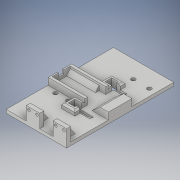
# Autodesk Inventor part: Elevator Slide
Saved by Autodesk Inventor 2018 (Build 220112000, 112)
## iProperties
Created: 2017-10-23
Part Number: Elevator Slide
Material: Generic
Document SubType Name: Modeling
Designer: thompson.nathaniel
Density: 1 g/cm^3
Appearance: Default
Author: thompson.nathaniel
Autodesk Inventor part; units mm, degrees
ref_plane "YZ Plane" through (0, 0, 0) normal (1, 0, 0) x (0, 1, 0)
ref_plane "XZ Plane" through (0, 0, 0) normal (0, 1, 0) x (-1, 0, 0)
ref_plane "XY Plane" through (0, 0, 0) normal (0, 0, 1) x (1, 0, 0)
sketch "Sketch1" plane through (0, 0, 0) normal (0, 1, 0) x (-1, 0, 0)
  line L0 (0, 0) -> (-114.3, 0)
  line L1 (-114.3, 0) -> (-114.3, 152.4)
  line L2 (-114.3, 152.4) -> (0, 152.4)
  line L3 (0, 152.4) -> (0, 0)
  line L4 (-69.85, 34.925) -> (-57.15, 34.925)
  line L5 (-57.15, 34.925) -> (-57.15, 47.625)
  line L6 (-57.15, 47.625) -> (-69.85, 47.625)
  line L7 (-69.85, 47.625) -> (-69.85, 34.925)
  line L8 (-69.85, 104.775) -> (-57.15, 104.775)
  line L9 (-57.15, 104.775) -> (-57.15, 117.475)
  line L10 (-57.15, 117.475) -> (-69.85, 117.475)
  line L11 (-69.85, 117.475) -> (-69.85, 104.775)
  dimension "d0" = 152.4
  dimension "d1" = 114.3
  dimension "d2" = 44.45
  dimension "d3" = 44.45
  dimension "d4" = 12.7
  dimension "d5" = 12.7
  dimension "d6" = 12.7
  dimension "d7" = 12.7
  dimension "d8" = 57.15
  dimension "d9" = 34.925
  constraints: 24 end point, 6 parallel, 3 horizontal, 3 perpendicular
  measures "d0" distance of L0.end L1.end
  measures "d1" distance of L0.start L0.end
  measures "d2" distance between parallel lines of L1 L7
  measures "d3" distance between parallel lines of L1 L11
  measures "d4" distance of L8.start L8.end
  measures "d5" distance of L10.end L8.start
  measures "d6" distance of L6.end L4.start
  measures "d7" distance of L4.start L4.end
  measures "d8" distance between parallel lines of L8 L6
  measures "d9" distance between parallel lines of L2 L10
extrude "Extrusion1" add sketch "Sketch1" along normal blind 10.16
sketch "Sketch2" plane through (0, 10.16, 0) normal (0, 1, 0) x (1, 0, 0)
  line L0 (50.8, -28.575) -> (76.2, -28.575)
  line L1 (76.2, -28.575) -> (76.2, -53.975)
  line L2 (76.2, -53.975) -> (50.8, -53.975)
  line L3 (50.8, -53.975) -> (50.8, -28.575)
  line L4 (50.8, -98.425) -> (76.2, -98.425)
  line L5 (76.2, -98.425) -> (76.2, -123.825)
  line L6 (76.2, -123.825) -> (50.8, -123.825)
  line L7 (50.8, -123.825) -> (50.8, -98.425)
  line L8 (57.15, -34.925) -> (69.85, -34.925) projected
  line L9 (69.85, -34.925) -> (69.85, -47.625) projected
  line L10 (69.85, -47.625) -> (57.15, -47.625) projected
  line L11 (57.15, -47.625) -> (57.15, -34.925) projected
  line L12 (57.15, -104.775) -> (69.85, -104.775) projected
  line L13 (69.85, -104.775) -> (69.85, -117.475) projected
  line L14 (69.85, -117.475) -> (57.15, -117.475) projected
  line L15 (57.15, -117.475) -> (57.15, -104.775) projected
  line L16 (57.15, -104.775) -> (57.15, -117.475)
  point P0 (0, 0)
  dimension "d12" = 6.35
  dimension "d13" = 6.35
  dimension "d14" = 6.35
  dimension "d15" = 6.35
  dimension "d16" = 6.35
  dimension "d17" = 6.35
  dimension "d18" = 6.35
  constraints: 18 end point, 5 equal length, 2 horizontal, 2 perpendicular, 1 point on line
  measures "d12" distance between parallel lines of L8 L0
  measures "d13" distance between parallel lines of L9 L1
  measures "d14" distance between parallel lines of L10 L2
  measures "d15" distance between parallel lines of L11 L3
  measures "d16" distance between parallel lines of L12 L4
  measures "d17" distance between parallel lines of L13 L5
  measures "d18" distance between parallel lines of L6 L14
extrude "Extrusion2" add sketch "Sketch2" along normal blind 8.89
chamfer "Chamfer1" distance 3.175 angle 45 8 edges at (63.5, 19.05, 123.825) (50.8, 19.05, 111.125) (63.5, 19.05, 98.425) (76.2, 19.05, 111.125) (63.5, 19.05, 53.975) (50.8, 19.05, 41.275) (63.5, 19.05, 28.575) (76.2, 19.05, 41.275)
sketch "Sketch3" plane through (0, 19.05, 0) normal (0, 1, 0) x (1, 0, 0)
  line L0 (69.85, -47.625) -> (69.85, -34.925) projected
  line L1 (76.2, -28.575) -> (76.2, -53.975) projected
  line L2 (69.85, -38.1) -> (76.2, -38.1)
  line L3 (76.2, -38.1) -> (76.2, -44.45)
  line L4 (76.2, -44.45) -> (69.85, -44.45)
  line L5 (69.85, -44.45) -> (69.85, -38.1)
  line L6 (69.85, -117.475) -> (69.85, -104.775) projected
  line L7 (76.2, -98.425) -> (76.2, -123.825) projected
  line L8 (69.85, -107.95) -> (76.2, -107.95)
  line L9 (76.2, -107.95) -> (76.2, -114.3)
  line L10 (76.2, -114.3) -> (69.85, -114.3)
  line L11 (69.85, -114.3) -> (69.85, -107.95)
  line L12 (57.15, -34.925) -> (69.85, -34.925) projected
  line L13 (69.85, -117.475) -> (57.15, -117.475) projected
  point P0 (0, 0)
  dimension "d24" = 6.35
  dimension "d25" = 3.175
  dimension "d26" = 3.175
  dimension "d27" = 6.35
  constraints: 16 end point, 4 parallel, 4 point on line, 2 horizontal, 2 perpendicular
  measures "d24" distance between parallel lines of L4 L2
  measures "d25" distance between parallel lines of L12 L2
  measures "d26" distance between parallel lines of L13 L10
  measures "d27" distance of L10.end L8.start
extrude "Extrusion3" cut sketch "Sketch3" against normal blind 8.89
sketch "Sketch4" plane through (0, 10.16, 0) normal (0, 1, 0) x (1, 0, 0)
  line L0 (69.85, -38.1) -> (88.9, -38.1)
  line L1 (88.9, -38.1) -> (88.9, -44.45)
  line L2 (88.9, -44.45) -> (69.85, -44.45)
  line L3 (69.85, -44.45) -> (69.85, -38.1)
  line L4 (69.85, -114.3) -> (69.85, -107.95) projected
  line L5 (69.85, -107.95) -> (95.25, -107.95)
  line L6 (95.25, -107.95) -> (95.25, -114.3)
  line L7 (95.25, -114.3) -> (69.85, -114.3)
  line L8 (69.85, -114.3) -> (69.85, -107.95)
  point P0 (0, 0)
  dimension "d30" = 25.4
  dimension "d31" = 6.35
  dimension "d32" = 6.35
  dimension "d33" = 19.05
  constraints: 16 end point, 4 parallel, 2 horizontal, 2 perpendicular
  measures "d30" distance of L6.end L7.end
  measures "d31" distance between parallel lines of L5 L7
  measures "d32" distance between parallel lines of L0 L2
  measures "d33" distance between parallel lines of L3 L1
extrude "Extrusion4" cut sketch "Sketch4" against normal blind 3.81
fillet "Fillet1" radius 21.336 2 edges at (88.9, 6.35, 41.275) (95.25, 6.35, 111.125)
sketch "Sketch5" plane through (0, 10.16, 0) normal (0, 1, 0) x (1, 0, 0)
  line L0 (0, -152.4) -> (0, 0) projected
  line L1 (0, -98.425) -> (100.33, -98.425)
  line L2 (100.33, -98.425) -> (100.33, -53.975)
  line L3 (100.33, -53.975) -> (0, -53.975)
  line L4 (0, -53.975) -> (0, -98.425)
  line L5 (50.8, -98.425) -> (76.2, -98.425) projected
  dimension "d37" = 44.45
  dimension "d38" = 0
  dimension "d39" = 100.33
  constraints: 8 end point, 2 parallel, 1 horizontal, 1 perpendicular, 1 point on line
  measures "d37" distance between parallel lines of L3 L1
  measures "d38" distance between parallel lines of L5 L1
  measures "d39" distance between parallel lines of L0 L2
extrude "Extrusion5" add sketch "Sketch5" along normal blind 12.7
sketch "Sketch6" plane through (100.33, 10.16, 98.425) normal (1, 0, 0) x (0, 0, -1)
  line L0 (44.45, 12.7) -> (0, 12.7) projected
  line L1 (5.08, 12.7) -> (5.08, 8.89)
  line L2 (5.08, 8.89) -> (11.811, 0)
  line L3 (44.45, 0) -> (0, 0) projected
  line L4 (32.639, 0) -> (39.37, 8.89)
  line L5 (39.37, 8.89) -> (39.37, 12.7)
  line L6 (5.08, 12.7) -> (39.37, 12.7)
  line L7 (0, 12.7) -> (44.45, 12.7) projected
  line L8 (0, 0) -> (0, 12.7) projected
  point P0 (98.425, -10.16)
  dimension "d42" = 34.29
  dimension "d43" = 5.08
  dimension "d44" = 20.828
  dimension "d45" = 8.89
  dimension "d46" = 8.89
  dimension "d47" = 6.731
  constraints: 10 end point, 4 point on line, 1 collinear, 1 parallel, 1 vertical
  measures "d42" distance between parallel lines of L5 L1
  measures "d43" distance between parallel lines of L8 L1
  measures "d44" distance of L4.start L2.end
  measures "d45" distance from line of L3 L1.end
  measures "d46" distance from line of L3 L4.end
  measures "d47" distance from line of L1 L2.end
extrude "Extrusion6" cut sketch "Sketch6" against normal blind 100.33 contours L5 L4 L3 L2 L1 L0
sketch "Sketch7" plane through (0, 22.86, 0) normal (0, 1, 0) x (1, 0, 0)
  line L0 (0, -98.425) -> (100.33, -98.425) projected
  line L1 (76.2, -53.975) -> (100.33, -53.975) projected
  line L2 (100.33, -98.425) -> (96.52, -98.425)
  line L3 (96.52, -98.425) -> (96.52, -53.975)
  line L4 (96.52, -53.975) -> (100.33, -53.975)
  line L5 (100.33, -53.975) -> (100.33, -98.425)
  point P0 (0, 0)
  dimension "d50" = 3.81
  constraints: 8 end point, 2 parallel, 1 horizontal, 1 perpendicular, 1 point on line
  measures "d50" distance between parallel lines of L5 L3
extrude "Extrusion7" add sketch "Sketch7" against normal blind 12.7
sketch "Sketch8" plane through (0, 22.86, 0) normal (0, 1, 0) x (1, 0, 0)
  line L0 (100.33, -98.425) -> (76.2, -98.425) projected
  line L1 (76.2, -53.975) -> (100.33, -53.975) projected
  line L2 (76.2, -98.425) -> (96.52, -98.425)
  line L3 (96.52, -98.425) -> (96.52, -53.975)
  line L4 (96.52, -53.975) -> (76.2, -53.975)
  line L5 (76.2, -53.975) -> (76.2, -98.425)
  point P0 (0, 0)
  constraints: 8 end point, 2 parallel, 1 horizontal, 1 perpendicular, 1 point on line
extrude "Extrusion8" cut sketch "Sketch8" against normal blind 12.7
sketch "Sketch9" plane through (100.33, 10.16, 98.425) normal (1, 0, 0) x (0, 0, -1)
  line L0 (0, 12.7) -> (44.45, 12.7) projected
  line L1 (44.45, 0) -> (0, 0) projected
  line L2 (0, 12.7) -> (44.45, 12.7)
  line L3 (44.45, 12.7) -> (44.45, 0)
  line L4 (44.45, 0) -> (0, 0)
  line L5 (0, 0) -> (0, 12.7)
  point P0 (98.425, -10.16)
  constraints: 8 end point, 2 parallel, 1 horizontal, 1 perpendicular
extrude "Extrusion9" add sketch "Sketch9" along normal blind 6.35
sketch "Sketch10" plane through (106.68, 10.16, 98.425) normal (1, 0, 0) x (0, 0, -1)
  line L0 (44.45, 0) -> (44.45, 12.7) projected
  line L1 (-25.4, 0) -> (0, 0) projected
  line L2 (44.45, 12.7) -> (0, 12.7)
  line L3 (0, 12.7) -> (0, 0)
  line L4 (0, 0) -> (44.45, 0)
  line L5 (44.45, 0) -> (44.45, 12.7)
  point P0 (98.425, -10.16)
  constraints: 8 end point, 2 parallel, 1 horizontal, 1 perpendicular
extrude "Extrusion10" add sketch "Sketch10" along normal blind 7.62
sketch "Sketch11" plane through (96.52, 22.86, 53.975) normal (-1, 0, 0) x (0, 0, 1)
  line L0 (0, -12.7) -> (0, 0) projected
  line L1 (44.45, 0) -> (44.45, -12.7) projected
  line L2 (0, -12.7) -> (44.45, -12.7)
  line L3 (44.45, -12.7) -> (44.45, 0)
  line L4 (44.45, 0) -> (0, 0)
  line L5 (0, 0) -> (0, -12.7)
  point P0 (-53.975, -22.86)
  constraints: 8 end point, 2 parallel, 1 horizontal, 1 perpendicular
extrude "Extrusion11" cut sketch "Sketch11" against normal blind 5.08
sketch "Sketch12" plane through (0, 22.86, 0) normal (0, 1, 0) x (1, 0, 0)
  line L0 (76.2, -59.055) -> (76.2, -53.975) projected
  line L1 (76.2, -93.345) -> (0, -93.345) projected
  line L2 (76.2, -59.055) -> (57.15, -59.055)
  line L3 (57.15, -59.055) -> (57.15, -93.345)
  line L4 (57.15, -93.345) -> (76.2, -93.345)
  line L5 (76.2, -93.345) -> (76.2, -59.055)
  line L6 (0, -93.345) -> (0, -98.425) projected
  point P0 (0, 0)
  dimension "d61" = 57.15
  constraints: 8 end point, 2 parallel, 1 horizontal, 1 perpendicular, 1 point on line
  measures "d61" distance between parallel lines of L6 L3
extrude "Extrusion12" cut sketch "Sketch12" against normal blind 12.7
sketch "Sketch13" plane through (101.6, 22.86, 53.975) normal (-1, 0, 0) x (0, 0, 1)
  line L0 (0, -12.7) -> (44.45, -12.7)
  line L1 (44.45, -12.7) -> (44.45, 0)
  line L2 (44.45, 0) -> (0, 0)
  line L3 (0, 0) -> (0, -12.7)
  point P0 (-53.975, -22.86)
  constraints: 8 end point, 2 parallel, 1 horizontal, 1 perpendicular
extrude "Extrusion13" cut sketch "Sketch13" along normal blind 31.75
sketch "Sketch14" plane through (69.85, 19.05, 107.95) normal (0, 0, 1) x (1, 0, 0)
  line L0 (6.35, -8.89) -> (25.4, -8.89) projected
  line L1 (0, 0) -> (6.35, 0)
  line L2 (6.35, 0) -> (6.35, -8.89)
  line L3 (6.35, -8.89) -> (0, -8.89)
  line L4 (0, -8.89) -> (0, 0)
  point P0 (-69.85, -19.05)
  dimension "d66" = 6.35
  dimension "d67" = 8.89
  constraints: 8 end point, 2 parallel, 1 horizontal, 1 perpendicular
  measures "d66" distance of L1.start L1.end
  measures "d67" distance of L1.end L0.start
extrude "Extrusion14" cut sketch "Sketch14" against normal blind 63.5
sketch "Sketch15" plane through (0, 10.16, 0) normal (0, 1, 0) x (1, 0, 0)
  circle A0 centre (20.32, -104.775) radius 3.81
  circle A1 centre (44.45, -104.775) radius 3.81
  circle A2 centre (20.32, -47.625) radius 3.81
  circle A3 centre (44.45, -47.625) radius 3.81
  line L0 (0, -98.425) -> (0, -152.4) projected
  line L1 (0, -53.975) -> (50.8, -53.975) projected
  line L2 (0, 0) -> (0, -53.975) projected
  line L3 (50.8, -98.425) -> (0, -98.425) projected
  dimension "d70" = 7.62
  dimension "d71" = 7.62
  dimension "d72" = 7.62
  dimension "d73" = 7.62
  dimension "d74" = 20.32
  dimension "d75" = 44.45
  dimension "d76" = 6.35
  dimension "d77" = 20.32
  dimension "d78" = 44.45
  dimension "d79" = 6.35
  dimension "d80" = 6.35
  dimension "d81" = 6.35
  constraints: 4 centre point
  measures "d70" diameter of A0
  measures "d71" diameter of A2
  measures "d72" diameter of A3
  measures "d73" diameter of A1
  measures "d74" distance from line of L0 A0.centre
  measures "d75" distance from line of L0 A1.centre
  measures "d76" distance from line of L1 A3.centre
  measures "d77" distance from line of L2 A2.centre
  measures "d78" distance from line of L2 A3.centre
  measures "d79" distance from line of L1 A2.centre
  measures "d80" distance from line of L3 A0.centre
  measures "d81" distance from line of L3 A1.centre
extrude "Extrusion15" cut sketch "Sketch15" against normal blind 10.16
sketch "Sketch16" plane through (0, 0, 152.4) normal (0, 0, 1) x (1, 0, 0)
  line L0 (57.15, 10.16) -> (0, 10.16) projected
  line L1 (114.3, 0) -> (0, 0) projected
  line L2 (0, 10.16) -> (114.3, 10.16)
  line L3 (114.3, 10.16) -> (114.3, 0)
  line L4 (114.3, 0) -> (0, 0)
  line L5 (0, 0) -> (0, 10.16)
  constraints: 8 end point, 2 parallel, 1 horizontal, 1 perpendicular
extrude "Extrusion16" add sketch "Sketch16" along normal blind 25.4
sketch "Sketch17" plane through (114.3, 0, 0) normal (0, 0, -1) x (-1, 0, 0)
  line L0 (114.3, 10.16) -> (114.3, 19.05) projected
  line L1 (0, 0) -> (0, 10.16) projected
  line L2 (114.3, 10.16) -> (0, 10.16)
  line L3 (0, 10.16) -> (0, 0)
  line L4 (0, 0) -> (114.3, 0)
  line L5 (114.3, 0) -> (114.3, 10.16)
  constraints: 8 end point, 2 parallel, 1 horizontal, 1 perpendicular
extrude "Extrusion17" add sketch "Sketch17" along normal blind 25.4
sketch "Sketch18" plane through (0, 0, 0) normal (0, -1, 0) x (1, 0, 0)
  line L0 (114.3, -25.4) -> (0, -25.4) projected
  line L1 (114.3, -25.4) -> (0, -25.4)
  line L2 (0, -25.4) -> (0, 177.8)
  line L3 (0, 177.8) -> (114.3, 177.8)
  line L4 (114.3, 177.8) -> (114.3, -25.4)
  line L5 (0, 177.8) -> (114.3, 177.8) projected
  point P0 (0, 0)
  dimension "d88" = 0
  dimension "d89" = 114.3
  constraints: 8 end point, 2 parallel, 1 horizontal, 1 perpendicular
  measures "d88" distance between parallel lines of L5 L3
  measures "d89" distance between parallel lines of L2 L4
extrude "Extrusion18" cut sketch "Sketch18" against normal blind 3.81
sketch "Sketch21" plane through (0, 3.81, 0) normal (0, -1, 0) x (1, 0, 0)
  circle A0 centre (71.12, 8.255) radius 3.81
  circle A1 centre (101.6, 8.255) radius 3.81
  line L0 (114.3, 177.8) -> (114.3, -25.4) projected
  point P0 (0, 0)
  point P1 (69.85, 59.055)
  point P2 (114.3, 176.403)
  point P3 (114.3, -24.003)
  dimension "d96" = 50.8
  dimension "d97" = 50.8
  dimension "d98" = 7.62
  dimension "d99" = 7.62
  dimension "d100" = 12.7
  dimension "d101" = 43.18
  constraints: 2 centre point
  measures "d96" vertical distance of point (69.85, 59.055) A0.centre
  measures "d97" vertical distance of A1.centre point (69.85, 59.055)
  measures "d98" diameter of A1
  measures "d99" diameter of A0
  measures "d100" distance from line of L0 A1.centre
  measures "d101" distance from line of L0 A0.centre
extrude "Extrusion21" cut sketch "Sketch21" against normal through all
sketch "Sketch22" plane through (0, 10.16, 0) normal (0, 1, 0) x (1, 0, 0)
  line L0 (114.3, -177.8) -> (114.3, 25.4) projected
  line L1 (114.3, -177.8) -> (88.9, -177.8)
  line L2 (88.9, -177.8) -> (88.9, -170.18)
  line L3 (88.9, -170.18) -> (114.3, -170.18)
  line L4 (114.3, -170.18) -> (114.3, -177.8)
  line L5 (114.3, -177.8) -> (0, -177.8) projected
  line L6 (63.5, -177.8) -> (38.1, -177.8)
  line L7 (38.1, -177.8) -> (38.1, -170.18)
  line L8 (38.1, -170.18) -> (63.5, -170.18)
  line L9 (63.5, -170.18) -> (63.5, -177.8)
  point P0 (0, 0)
  dimension "d104" = 25.4
  dimension "d105" = 25.4
  dimension "d106" = 25.4
  dimension "d107" = 7.62
  constraints: 16 end point, 4 parallel, 2 horizontal, 2 perpendicular, 2 point on line
  measures "d104" distance of L7.end L8.end
  measures "d105" distance between parallel lines of L2 L9
  measures "d106" distance of L0.start L1.end
  measures "d107" distance between parallel lines of L5 L8
extrude "Extrusion22" add sketch "Sketch22" along normal blind 25.4
sketch "Sketch23" plane through (0, 10.16, 0) normal (0, 1, 0) x (1, 0, 0)
  line L0 (38.1, -170.18) -> (63.5, -170.18) projected
  line L1 (46.99, -170.18) -> (54.61, -170.18)
  line L2 (54.61, -170.18) -> (54.61, -152.4)
  line L3 (54.61, -152.4) -> (46.99, -152.4)
  line L4 (46.99, -152.4) -> (46.99, -170.18)
  line L5 (97.79, -170.18) -> (105.41, -170.18)
  line L6 (105.41, -170.18) -> (105.41, -152.4)
  line L7 (105.41, -152.4) -> (97.79, -152.4)
  line L8 (97.79, -152.4) -> (97.79, -170.18)
  line L9 (38.1, -170.18) -> (38.1, -177.8) projected
  line L10 (88.9, -170.18) -> (88.9, -177.8) projected
  point P0 (0, 0)
  dimension "d110" = 7.62
  dimension "d111" = 8.89
  dimension "d112" = 8.89
  dimension "d113" = 7.62
  dimension "d114" = 17.78
  dimension "d115" = 17.78
  constraints: 16 end point, 4 parallel, 2 horizontal, 2 perpendicular, 2 point on line
  measures "d110" distance between parallel lines of L4 L2
  measures "d111" distance between parallel lines of L9 L4
  measures "d112" distance between parallel lines of L10 L8
  measures "d113" distance between parallel lines of L8 L6
  measures "d114" distance between parallel lines of L5 L7
  measures "d115" distance between parallel lines of L0 L3
extrude "Extrusion23" add sketch "Sketch23" along normal blind 25.4
chamfer "Chamfer2" distance 17.78 distance2 25.4 1 edges at (101.6, 35.56, 152.4) measured on face at (100.33, 35.56, 175.26)
chamfer "Chamfer3" distance 17.78 distance2 25.4 1 edges at (50.8, 35.56, 152.4) measured on face at (49.53, 35.56, 175.26)
sketch "Sketch24" plane through (114.3, 10.16, 170.18) normal (0, 0, -1) x (-1, 0, 0)
  circle A0 centre (5.08, 20.32) radius 2.54
  circle A1 centre (20.32, 20.32) radius 2.54
  circle A2 centre (55.88, 20.32) radius 2.54
  circle A3 centre (71.12, 20.32) radius 2.54
  line L0 (16.51, 25.4) -> (25.4, 25.4) projected
  line L1 (25.4, 0) -> (25.4, 25.4) projected
  line L2 (0, 25.4) -> (8.89, 25.4) projected
  line L3 (0, 0) -> (0, 25.4) projected
  line L4 (50.8, 0) -> (50.8, 25.4) projected
  line L5 (67.31, 25.4) -> (76.2, 25.4) projected
  line L6 (76.2, 0) -> (76.2, 25.4) projected
  line L7 (50.8, 25.4) -> (59.69, 25.4) projected
  point P0 (114.3, -10.16)
  dimension "d124" = 5.08
  dimension "d125" = 5.08
  dimension "d126" = 5.08
  dimension "d127" = 5.08
  dimension "d128" = 5.08
  dimension "d129" = 5.08
  dimension "d130" = 5.08
  dimension "d131" = 5.08
  dimension "d132" = 5.08
  dimension "d133" = 5.08
  dimension "d134" = 5.08
  dimension "d135" = 5.08
  constraints: 4 centre point
  measures "d124" diameter of A0
  measures "d125" diameter of A2
  measures "d126" diameter of A3
  measures "d127" diameter of A1
  measures "d128" distance from line of L0 A1.centre
  measures "d129" distance from line of L1 A1.centre
  measures "d130" distance from line of L2 A0.centre
  measures "d131" distance from line of L3 A0.centre
  measures "d132" distance from line of L4 A2.centre
  measures "d133" distance from line of L5 A3.centre
  measures "d134" distance from line of L6 A3.centre
  measures "d135" distance from line of L7 A2.centre
extrude "Extrusion24" cut sketch "Sketch24" against normal blind 25.4
sketch "Sketch25" plane through (101.6, 22.86, 53.975) normal (-1, 0, 0) x (0, 0, 1)
  line L0 (0, -12.7) -> (0, 0) projected
  line L1 (0, 0) -> (44.45, 0) projected
  line L2 (0, -12.7) -> (44.45, -12.7)
  line L3 (44.45, -12.7) -> (44.45, 0)
  line L4 (44.45, 0) -> (0, 0)
  line L5 (0, 0) -> (0, -12.7)
  point P0 (-53.975, -22.86)
  constraints: 8 end point, 2 parallel, 1 horizontal, 1 perpendicular
extrude "Extrusion25" add sketch "Sketch25" along normal blind 3.0734
sketch "Sketch26" plane through (0, 10.16, 0) normal (0, 1, 0) x (1, 0, 0)
  line L0 (98.5266, -53.975) -> (83.2866, -53.975)
  line L1 (83.2866, -53.975) -> (83.2866, -98.425)
  line L2 (83.2866, -98.425) -> (98.5266, -98.425)
  line L3 (98.5266, -98.425) -> (98.5266, -53.975)
  line L4 (114.3, -98.425) -> (98.5266, -98.425) projected
  point P0 (0, 0)
  dimension "d140" = 0
  dimension "d141" = 15.24
  constraints: 8 end point, 2 parallel, 1 horizontal, 1 perpendicular
  measures "d140" distance between parallel lines of L4 L2
  measures "d141" distance between parallel lines of L3 L1
extrude "Extrusion26" add sketch "Sketch26" along normal blind 12.954
chamfer "Chamfer4" distance 15.24 distance2 12.954 1 edges at (83.2866, 23.114, 76.2) measured on face at (93.4466, 23.114, 83.6083)
sketch "Sketch27" plane through (0, 22.86, 0) normal (0, 1, 0) x (1, 0, 0)
  line L0 (98.5266, -98.425) -> (98.5266, -53.975) projected
  line L1 (98.5266, -53.975) -> (114.3, -53.975) projected
  line L2 (98.5266, -98.425) -> (114.3, -98.425)
  line L3 (114.3, -98.425) -> (114.3, -53.975)
  line L4 (114.3, -53.975) -> (98.5266, -53.975)
  line L5 (98.5266, -53.975) -> (98.5266, -98.425)
  point P0 (0, 0)
  constraints: 8 end point, 2 parallel, 1 horizontal, 1 perpendicular
extrude "Extrusion27" add sketch "Sketch27" along normal blind 0.254
sketch "Sketch28" plane through (0, 22.86, 0) normal (0, 1, 0) x (1, 0, 0)
  line L0 (0, -93.345) -> (0, -98.425) projected
  line L1 (69.85, -53.975) -> (0, -53.975) projected
  line L2 (0, -98.425) -> (2.54, -98.425)
  line L3 (2.54, -98.425) -> (2.54, -53.975)
  line L4 (2.54, -53.975) -> (0, -53.975)
  line L5 (0, -53.975) -> (0, -98.425)
  point P0 (0, 0)
  dimension "d149" = 2.54
  constraints: 8 end point, 2 parallel, 1 horizontal, 1 perpendicular, 1 point on line
  measures "d149" distance between parallel lines of L5 L3
extrude "Extrusion28" add sketch "Sketch28" against normal blind 12.7
sketch "Sketch29" plane through (2.54, 22.86, 93.345) normal (1, 0, 0) x (0, 0, -1)
  line L0 (12.065, -6.858) -> (22.225, -6.858)
  line L1 (22.225, -6.858) -> (22.225, 0)
  line L2 (22.225, 0) -> (12.065, 0)
  line L3 (12.065, 0) -> (12.065, -6.858)
  line L4 (27.559, -12.7) -> (6.731, -12.7) projected
  line L5 (0, 0) -> (34.29, 0) projected
  point P0 (93.345, -22.86)
  dimension "d152" = 5.842
  dimension "d153" = 5.334
  dimension "d154" = 5.334
  dimension "d155" = 0
  constraints: 8 end point, 2 parallel, 1 horizontal, 1 perpendicular
  measures "d152" distance between parallel lines of L4 L0
  measures "d153" distance from line of L4.start L1
  measures "d154" distance from line of L4.end L3
  measures "d155" distance between parallel lines of L2 L5
extrude "Extrusion29" cut sketch "Sketch29" against normal blind 12.7
body "Solid1"
